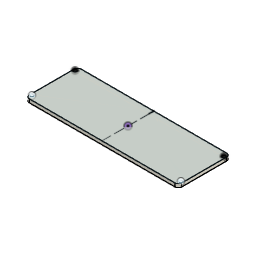
Upper Level Mount - Blank (Autodesk Fusion 360 design; units mm, degrees)
Autodesk Fusion 360 part; units mm, degrees
sketch "Sketch1" plane through (0, 0, 0) normal (0, 0, 1) x (-1, 0, 0)
  line L0 (-88.5, 30) -> (88.5, 30)
  line L1 (88.5, 30) -> (88.5, -30)
  line L2 (88.5, -30) -> (-88.5, -30)
  line L3 (-88.5, -30) -> (-88.5, 30)
  point P0 (0, 30)
  point P1 (-88.5, 0)
  dimension "d44_2_2" = 177
  dimension "d45_2_2" = 60
  dimension "d54_2_2" = 30
  dimension "d55_2_2" = 87.5
  constraint horizontal L0
  constraint vertical L1
  constraint horizontal L2
  constraint vertical L3
  constraint midpoint L0 P0
  constraint midpoint L3 P1
  constraint vertical origin P0
  constraint horizontal origin P1
  measures "d44_2_2" distance of L0.start L0.end
  measures "d45_2_2" distance of L0.start L2.end
  measures "d54_2_2" distance of L0.start P1
extrude "Extrude1" add sketch "Sketch1" along normal blind 4
fillet "Fillet1" radius 4 4 edges at (88.5, 30, 2) (88.5, -30, 2) (-88.5, 30, 2) (-88.5, -30, 2)
sketch "Sketch3" plane through (0, 0, 4) normal (0, 0, 1) x (-1, 0, 0)
  arc A0 (88.5, 26) -> (84.5, 30) centre (84.5, 26) ccw
  line L0 (84.5, 30) -> (-84.5, 30)
  arc A1 (-84.5, 30) -> (-88.5, 26) centre (-84.5, 26) ccw
  line L1 (-88.5, 26) -> (-88.5, -26)
  arc A2 (-88.5, -26) -> (-84.5, -30) centre (-84.5, -26) ccw
  line L2 (-84.5, -30) -> (84.5, -30)
  arc A3 (84.5, -30) -> (88.5, -26) centre (84.5, -26) ccw
  line L3 (88.5, -26) -> (88.5, 26)
  line L4 (0, -30) -> (0, -24.8801)
  line L5 (0, -24.8801) -> (0, 30) construction
  circle A4 centre (86.5, -25) radius 1.7
  circle A5 centre (86.5, 25) radius 1.7
  circle A6 centre (-86.5, -25) radius 1.7
  circle A7 centre (-86.5, 25) radius 1.7
  dimension "d56_2_2" = 3.4
  dimension "d57_2_2" = 3.4
  dimension "d58_2_2" = 3.4
  dimension "d59_2_2" = 3.4
  dimension "d61_2_2" = 5
  dimension "d105_1_2" = 50
  dimension "d6" = 171
  constraint midpoint L2 L4.start
  constraint midpoint L0 L5.end
  constraint horizontal A4.centre A6.centre
  constraint vertical A6.centre A7.centre
  constraint horizontal A5.centre A7.centre
  constraint vertical A4.centre A5.centre
  constraint symmetric L5 A4.centre A6.centre
  measures "d56_2_2" diameter of A4
  measures "d57_2_2" diameter of A6
  measures "d58_2_2" diameter of A5
  measures "d59_2_2" diameter of A7
  measures "d61_2_2" distance of L2 A4.centre
  measures "d105_1_2" distance of A4.centre A5.centre
  measures "d6" horizontal distance of A2.centre A4.centre
extrude "Extrude3" cut sketch "Sketch3" against normal through all contours A4 | A5 | A6 | A7
equation "d57_2_2 = d56_2_2"
equation "d58_2_2 = d56_2_2"
equation "d59_2_2 = d56_2_2"
